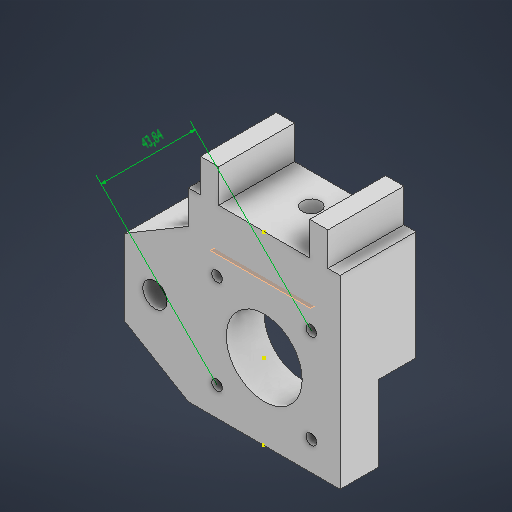
# Autodesk Inventor part: SuporteMotor
Saved by Autodesk Inventor 2026.1 (Build 301233000, 233)
## iProperties
Created: 2026-01-23
Part Number: SuporteMotor
Material: Generic
Document SubType Name: Modeling
Designer: fheli
Density: 1 g/cm^3
Appearance: Default
Author: fheli
Autodesk Inventor part; units mm, degrees
ref_plane "YZ Plane" through (0, 0, 0) normal (1, 0, 0) x (0, 1, 0)
ref_plane "XZ Plane" through (0, 0, 0) normal (0, 1, 0) x (-1, 0, 0)
ref_plane "XY Plane" through (0, 0, 0) normal (0, 0, 1) x (1, 0, 0)
sketch "Sketch1" plane through (0, 0, 0) normal (0, 0, 1) x (1, 0, 0)
  point P0 (0, 0)
sketch "Sketch2" plane through (0, 0, 0) normal (0, 0, 1) x (1, 0, 0)
  line L0 (-25, -25) -> (25, -25)
  line L1 (25, -25) -> (25, 25)
  circle A0 centre (0, 0) radius 12.5
  circle A1 centre (-15.5, 15.5) radius 1.75
  line L2 (25, 25) -> (25, 19)
  line L3 (25, -25) -> (19, -25)
  line L4 (-25, -25) -> (-19, -25)
  circle A2 centre (-15.5, -15.5) radius 1.75
  circle A3 centre (15.5, -15.5) radius 1.75
  circle A4 centre (15.5, 15.5) radius 1.75
  line L5 (-25, 25) -> (-25, 36)
  line L6 (25, 36) -> (25, 25)
  line L7 (0, 36) -> (15, 36)
  line L8 (15, 36) -> (15, 47)
  line L9 (15, 47) -> (21, 47)
  line L10 (21, 47) -> (21, 36)
  line L11 (0, 36) -> (-15, 36)
  line L12 (-15, 36) -> (-15, 47)
  line L13 (-15, 47) -> (-21, 47)
  line L14 (-21, 47) -> (-21, 36)
  circle A5 centre (-36, 0) radius 4
  line L15 (-46, 0) -> (-46, 12.5)
  line L16 (-46, 12.5) -> (-25, 25)
  line L17 (-46, 0) -> (-46, -12.5)
  line L18 (-46, -12.5) -> (-25, -25)
  line L19 (-25, 36) -> (-21, 36)
  line L20 (-15, 36) -> (15, 36)
  line L21 (21, 36) -> (25, 36)
  line L22 (-21, -21) -> (21, -21)
  line L23 (21, -21) -> (21, 21)
  line L24 (21, 21) -> (-21, 21)
  line L25 (-21, 21) -> (-21, -21)
  line L26 (-21, -21) -> (21, 21) construction
  line L27 (21, -21) -> (-21, 21) construction
  dimension "d1" = 50
  dimension "d2" = 25
  dimension "d14" = 3.5
  dimension "d15" = 11
  dimension "d18" = 11
  dimension "d69" = 42
  dimension "d70" = 42
  dimension "d71" = 5.5
  dimension "d72" = 5.5
  dimension "d73" = 5.5
  dimension "d74" = 5.5
  dimension "d75" = 5.5
  dimension "d76" = 5.5
  dimension "d77" = 5.5
  dimension "d78" = 5.5
  dimension "d79" = 8
  dimension "d87" = 36
  dimension "d88" = 46
  dimension "d89" = 25
  dimension "d90" = 50
  dimension "d91" = 50
  dimension "d92" = 15
  dimension "d93" = 6
  dimension "d94" = 4
  constraints: 56 end point, 17 perpendicular, 6 centre point, 4 midpoint, 3 point on line, 3 vertical, 2 horizontal, 2 parallel, 1 coincident
  measures "d1" distance of L1.end L0.end
  measures "d2" diameter of A0
  measures "d14" diameter of A4
  measures "d15" distance of L5.start L5.end
  measures "d18" distance of L7.end L8.end
  measures "d69" distance of L24.end L23.end
  measures "d70" distance of L23.end L22.end
  measures "d71" distance from line of L23 A4.centre
  measures "d72" distance from line of L24 A4.centre
  measures "d73" distance from line of L24 A1.centre
  measures "d74" distance from line of L25 A1.centre
  measures "d75" distance from line of L23 A3.centre
  measures "d76" distance from line of L22 A3.centre
  measures "d77" distance from line of L22 A2.centre
  measures "d78" distance from line of L25 A2.centre
  measures "d79" diameter of A5
  measures "d87" distance of A5.centre point (0, 0)
  measures "d88" distance from line of L15 point (0, 0)
  measures "d89" distance of L15.end L17.end
  measures "d90" distance of L5.start L0.start
  measures "d91" distance of L0.end L0.start
  measures "d92" distance of L7.end point (0, 36)
  measures "d93" distance of L12.end L13.end
  measures "d94" distance of L5.end L14.end
extrude "Extrusion1" add sketch "Sketch2" against normal blind 25 contours L18 L17 L15 L16 L5 L19 L14 L13 L12 L11 L7 L8 L9 L10 L21 L6 L1 L0 | L25 L24 L23 L22
sketch "Sketch3" plane through (0, 0, 0) normal (0, 1, 0) x (-1, 0, 0)
  point P0 (0, 0)
sketch "Sketch4" plane through (-25, -25, 0) normal (0, -1, 0) x (1, 0, 0)
  point P0 (25, 0)
sketch "Sketch6" plane through (-25, -25, 0) normal (0, -1, 0) x (1, 0, 0)
  line L0 (50, -25) -> (-21, -25)
  line L1 (-21, -25) -> (-21, -12.5)
  line L2 (-21, -12.5) -> (50, -12.5)
  line L3 (50, -12.5) -> (50, -25)
  point P0 (25, 0)
  dimension "d34" = 71
  dimension "d35" = 12.5
  constraints: 8 end point, 2 parallel, 1 horizontal, 1 perpendicular
  measures "d34" distance of L1.end L2.end
  measures "d35" distance of L0.end L1.end
extrude "Extrusion2" cut sketch "Sketch6" against normal blind 25
sketch "Sketch7" plane through (25, -25, -12.5) normal (0, 0, -1) x (-1, 0, 0)
  circle A0 centre (40.5, 9.5) radius 1.75 projected
  circle A1 centre (40.5, 9.5) radius 3
  point P0 (25, 25)
  dimension "d38" = 6
  constraints: 1 centre point, 1 coincident
  measures "d38" diameter of A1
extrude "Extrusion3" cut sketch "Sketch7" against normal blind 4 contours A0 | A1
sketch "Sketch8" plane through (25, -25, -12.5) normal (0, 0, -1) x (-1, 0, 0)
  circle A0 centre (9.5, 9.5) radius 1.75 projected
  circle A1 centre (9.5, 9.5) radius 3
  point P0 (25, 25)
  dimension "d44" = 6
  constraints: 1 centre point, 1 coincident
  measures "d44" diameter of A1
extrude "Extrusion4" cut sketch "Sketch8" against normal blind 4 contours A0 | A1
sketch "Sketch9" plane through (0, 0, -25) normal (0, 0, -1) x (-1, 0, 0)
  circle A0 centre (15.5, 15.5) radius 1.75 projected
  circle A1 centre (15.5, 15.5) radius 3
  circle A2 centre (-15.5, 15.5) radius 1.75 projected
  circle A3 centre (-15.5, 15.5) radius 3
  point P0 (0, 0)
  dimension "d47" = 6
  dimension "d48" = 6
  constraints: 2 centre point, 2 coincident
  measures "d47" diameter of A1
  measures "d48" diameter of A3
extrude "Extrusion5" cut sketch "Sketch9" against normal blind 5 contours A1
sketch "Sketch10" plane through (0, 0, -25) normal (0, 0, -1) x (-1, 0, 0)
  circle A0 centre (-15.5, 15.5) radius 1.75 projected
  circle A1 centre (-15.5, 15.5) radius 3
  point P0 (0, 0)
  dimension "d51" = 6
  constraints: 1 centre point, 1 coincident
  measures "d51" diameter of A1
extrude "Extrusion6" cut sketch "Sketch10" against normal blind 5 contours A0 | A1
move faces "Move1" translate (0, 0, -12.5) faces at (-4.8121, -22.7683, -12.5)
sketch "Sketch11" plane through (-25, -25, 0) normal (0, -1, 0) x (1, 0, 0)
  line L0 (0, -25) -> (50, -25) projected
  line L1 (50, -25) -> (-21, -25)
  line L2 (-21, -25) -> (-21, -12.5)
  line L3 (-21, -12.5) -> (50, -12.5)
  line L4 (50, -12.5) -> (50, -25)
  point P0 (25, 0)
  dimension "d60" = 71
  dimension "d61" = 12.5
  constraints: 8 end point, 2 parallel, 1 horizontal, 1 perpendicular
  measures "d60" distance of L2.end L3.end
  measures "d61" distance of L1.end L2.end
extrude "Extrusion7" cut sketch "Sketch11" against normal blind 15
sketch "Sketch12" plane through (-25, -10, 0) normal (0, -1, 0) x (1, 0, 0)
  line L0 (50, -12.5) -> (50, -25) projected
  line L1 (50, -25) -> (0, -25)
  line L2 (0, -25) -> (0, -12.5)
  line L3 (0, -12.5) -> (50, -12.5)
  line L4 (50, -12.5) -> (50, -25)
  point P0 (25, 0)
  dimension "d64" = 50
  dimension "d65" = 12.5
  constraints: 8 end point, 2 parallel, 1 horizontal, 1 perpendicular
  measures "d64" distance of L2.end L3.end
  measures "d65" distance of L1.end L2.end
extrude "Extrusion8" cut sketch "Sketch12" against normal blind 10
sketch "Sketch13" plane through (-15, 36, 0) normal (0, 1, 0) x (1, 0, 0)
  point P0 (15, 0)
sketch "Sketch14" plane through (-15, 36, 0) normal (0, 1, 0) x (1, 0, 0)
  circle A0 centre (15.5463, 15) radius 3
  point P0 (15, 0)
  dimension "d80" = 6
  constraints: 1 centre point
  measures "d80" diameter of A0
extrude "Extrusion9" cut sketch "Sketch14" against normal blind 25
ref_plane "Work Plane6" through (-15, 23, 0) normal (0, 1, 0) x (1, 0, 0)
sketch "Sketch15" plane through (-15, 23, 0) normal (0, 1, 0) x (1, 0, 0)
  circle A0 centre (15.5858, 15.0671) radius 5.75
  point P0 (15, 0)
  dimension "d84" = 11.5
  constraints: 1 centre point
  measures "d84" diameter of A0
extrude "Extrusion10" cut sketch "Sketch15" against normal blind 25
body "Solid1"
